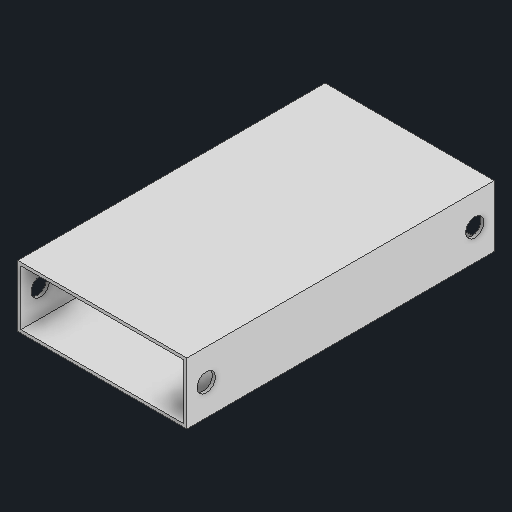
# Autodesk Inventor part: 铝方管
Saved by Autodesk Inventor 2025 (Build 290162000, 162)
## iProperties
Created: 2026-01-01
Part Number: 铝方管
Material: 常规
Document SubType Name: Modeling
Designer: XH
Density: 1 g/cm^3
Appearance: 默认
Author: XH
Autodesk Inventor part; units mm, degrees
ref_plane "YZ Plane" through (0, 0, 0) normal (1, 0, 0) x (0, 1, 0)
ref_plane "XZ Plane" through (0, 0, 0) normal (0, 1, 0) x (-1, 0, 0)
ref_plane "XY Plane" through (0, 0, 0) normal (0, 0, 1) x (1, 0, 0)
sketch "草图1" plane through (0, 0, 0) normal (0, 0, 1) x (1, 0, 0)
  line L0 (27.5, -10) -> (-27.5, -10)
  line L1 (-27.5, -10) -> (-27.5, 10)
  line L2 (-27.5, 10) -> (27.5, 10)
  line L3 (27.5, 10) -> (27.5, -10)
  line L4 (27.5, -10) -> (-27.5, 10) construction
  line L5 (-27.5, -10) -> (27.5, 10) construction
  point P0 (0, 0)
  dimension "d0" = 55
  dimension "d1" = 20
  constraints: 12 end point, 2 midpoint, 2 parallel, 1 horizontal, 1 perpendicular
  measures "d0" distance of L1.end L2.end
  measures "d1" distance of L0.end L1.end
extrude "拉伸1" add sketch "草图1" along normal blind 100
sketch "草图2" plane through (0, 0, 0) normal (0, 0, -1) x (-1, 0, 0)
  line L0 (-27.5, 10) -> (27.5, 10) projected
  line L1 (-27.5, -10) -> (-27.5, 10) projected
  line L2 (27.5, -10) -> (-27.5, -10) projected
  line L3 (27.5, 10) -> (27.5, -10) projected
  line L4 (26.5, -9) -> (-26.5, -9)
  line L5 (-26.5, -9) -> (-26.5, 9)
  line L6 (-26.5, 9) -> (26.5, 9)
  line L7 (26.5, 9) -> (26.5, -9)
  point P0 (0, 0)
  dimension "d4" = 1
  constraints: 8 end point, 3 other
  measures "d4" distance between parallel lines of L3 L7
extrude "拉伸2" cut sketch "草图2" against normal blind 109.25 contours L4 L5 L6 L7
sketch "草图3" plane through (-27.5, -10, 0) normal (-1, 0, 0) x (0, 0, 1)
  line L0 (100, 19) -> (100, 1) projected
  line L1 (100, 10) -> (53.3489, 10)
  circle A0 centre (93.6894, 10) radius 3
  point P0 (0, 10)
  dimension "d7" = 6
  constraints: 2 end point, 1 centre point, 1 horizontal, 1 midpoint, 1 point on line
  measures "d7" diameter of A0
extrude "拉伸3" cut sketch "草图3" against normal blind 109.25
ref_plane "工作平面1" through (0, 0, 50) normal (0, 0, -1) x (-1, 0, 0)
mirror "镜像1" about plane through (0, 0, 50) normal (0, 0, -1) of "拉伸3"
